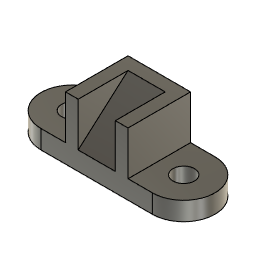
A2 (Autodesk Fusion 360 design; units mm, degrees)
Autodesk Fusion 360 part; units mm, degrees
sketch "Sketch1" plane through (0, 0, 0) normal (0, 0, 1) x (1, 0, 0)
  line L0 (57, 32) -> (-57, 32)
  line L1 (-57, -32) -> (57, -32)
  circle A0 centre (57, 0) radius 11
  circle A1 centre (-57, 0) radius 11
  arc A2 (-57, 32) -> (-57, -32) centre (-57, 0) ccw
  arc A3 (57, -32) -> (57, 32) centre (57, 0) ccw
  constraint horizontal L0
  constraint parallel L0 L1
  constraint concentric A0 A3
  constraint concentric A1 A2
extrude "Extrude1" add sketch "Sketch1" along normal blind 19
sketch "Sketch2" plane through (0, 0, 19) normal (0, 0, 1) x (-1, 0, 0)
  circle A0 centre (-57, 0) radius 11
  circle A1 centre (57, 0) radius 11
  arc A2 (-57, 32) -> (-57, -32) centre (-57, 0) ccw
  line L0 (-57, -32) -> (57, -32)
  arc A3 (57, -32) -> (57, 32) centre (57, 0) ccw
  line L1 (57, 32) -> (-57, 32)
  line L2 (32, 32) -> (32, -32)
  line L3 (-32, 32) -> (-32, -32)
  line L4 (32, -32) -> (-32, -32)
  line L5 (19, 32) -> (19, -19)
  line L6 (-19, 32) -> (-19, -19)
  line L7 (19, -19) -> (-19, -19)
  line L8 (32, 32) -> (19, 32)
  line L9 (-19, 32) -> (-32, 32)
  constraint coincident L1 L2.start
  constraint coincident L0 L2.end
  constraint perpendicular L0 L2
  constraint coincident L1 L3.start
  constraint coincident L0 L3.end
  constraint perpendicular L0 L3
  constraint coincident L1 L5.start
  constraint coincident L1 L6.start
  constraint perpendicular L1 L5
  constraint perpendicular L1 L6
  constraint perpendicular L6 L7
extrude "Extrude2" add sketch "Sketch2" along normal blind 45 contours L0 L1 L2 L3 L4 L5 L6 L7 L8 L9
sketch "Sketch3" plane through (19, 0, 0) normal (-1, 0, 0) x (0, -1, 0)
  line L0 (-19, 19) -> (32, 19)
  line L1 (32, 19) -> (32, 64)
  line L2 (32, 64) -> (-19, 64)
  line L3 (-19, 64) -> (-19, 19)
  line L4 (-19, 64) -> (32, 19)
  line L5 (-19, 64) -> (-19, 19)
  constraint coincident L2.end L3.start
  constraint coincident L0.end L1.start
  constraint coincident L0.start L3.end
extrude "Extrude3" add sketch "Sketch3" along normal blind 38 contours L0 L3 L4 L5
